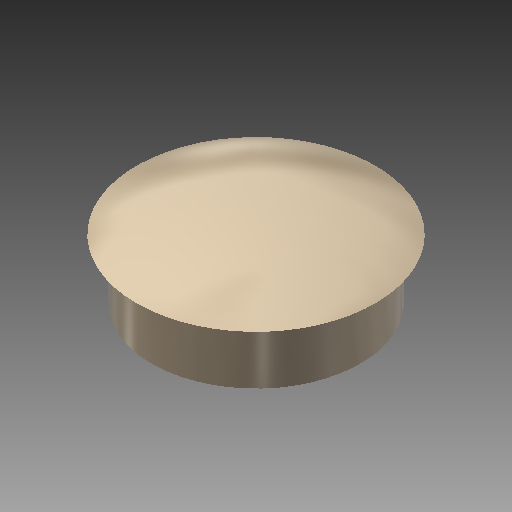
# Autodesk Inventor part: Zaślepka_do_rur_fi32
Saved by Autodesk Inventor 2017 (Build 210142000, 142)
## iProperties
Created: 2016-01-13
Part Number: Zaślepka_do_rur_fi32
Material: Polietylen o dużej gęstości
Document SubType Name: Modeling
Designer: graaapsik
Density: 0.952 g/cm^3
Appearance: Gładki - w kolorze złamanej bieli
Mass: 1.80794 g
Surface Area: 29.9394 cm^2
Volume: 1.89909 cm^3
Author: graaapsik
Autodesk Inventor part; units mm, degrees
ref_plane "YZ Plane" through (0, 0, 0) normal (1, 0, 0) x (0, 1, 0)
ref_plane "XZ Plane" through (0, 0, 0) normal (0, 1, 0) x (-1, 0, 0)
ref_plane "XY Plane" through (0, 0, 0) normal (0, 0, 1) x (1, 0, 0)
sketch "Szkic1" plane through (0, 0, 0) normal (0, 1, 0) x (-1, 0, 0)
  circle A0 centre (0, 0) radius 14
  dimension "d0" = 28
  constraints: 1 centre point, 1 coincident
  measures "d0" diameter of A0
extrude "Wyciągnięcie proste1" add sketch "Szkic1" along normal blind 8
shell "Skorupa1" thickness 1 removed faces 2 at (-0.5625, 0, 1.5565) at (-0.5625, 8, 1.5565)
sketch "Szkic2" plane through (0, 0, 0) normal (1, 0, 0) x (0, 1, 0)
  line L0 (8, -14) -> (8, 14) construction
  line L1 (8, 0) -> (11, 0)
  line L2 (8, 0) -> (8, 16)
  arc A0 (11, 0) -> (8, 16) centre (-33.1667, 0) ccw
  point P0 (0, 0)
  dimension "d4" = 3
  dimension "d5" = 16
  constraints: 4 end point, 2 perpendicular, 2 point on circle, 1 centre point, 1 line through centre, 1 midpoint
  measures "d4" distance of L1.start L1.end
  measures "d5" distance of L1.start L2.end
revolve "Obrót1" add sketch "Szkic2" angle 360 about axis through (0, 8, 0) along (0, 1, 0)
